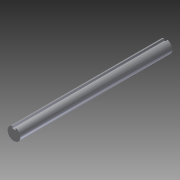
# Autodesk Inventor part: .5in diameter keyed axle
Saved by Autodesk Inventor 2011 SP1 (Build 150282100, 282)
## iProperties
Created: 2013-01-18
Part Number: .5in diameter keyed axle
Document SubType Name: Modeling
Designer: wes
Density: 1 g/cm^3
Author: wes
Autodesk Inventor part; units mm, degrees
ref_plane "YZ Plane" through (0, 0, 0) normal (1, 0, 0) x (0, 1, 0)
ref_plane "XZ Plane" through (0, 0, 0) normal (0, 1, 0) x (-1, 0, 0)
ref_plane "XY Plane" through (0, 0, 0) normal (0, 0, 1) x (1, 0, 0)
sketch "Sketch1" plane through (0, 0, 0) normal (0, 0, 1) x (1, 0, 0)
  circle A0 centre (0, 0) radius 6.35
  line L0 (-1.6002, 6.1451) -> (-1.6002, 3.8845)
  line L1 (-1.6002, 3.8845) -> (1.6002, 3.8845)
  line L2 (1.6002, 3.8845) -> (1.6002, 6.1451)
  line L3 (0, 0) -> (0, 7.6821)
  dimension "d0" = 12.7
  dimension "d1" = 3.2004
  dimension "d2" = 1.6002
  dimension "d3" = 2.2606
  constraints: 8 end point, 2 parallel, 2 point on circle, 1 centre point, 1 coincident, 1 perpendicular, 1 vertical
  measures "d0" diameter of A0
  measures "d1" distance of L0.end L1.end
  measures "d2" distance between parallel lines of L2 L3
  measures "d3" distance of L0.start L0.end
extrude "Extrusion1" add sketch "Sketch1" along normal blind 152.4 contours A0 L0 L1 L2
body "Solid1"
